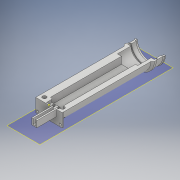
# Autodesk Inventor part: ExtendedHousingSide2wWireSupport
Saved by Autodesk Inventor 2019 (Build 230136000, 136)
## iProperties
Created: 2017-03-28
Part Number: ExtendedHousingSide2wWireSupport
Material: Generic
Document SubType Name: Modeling
Designer: Joseph
Density: 1 g/cm^3
Appearance: Default
Author: Joseph
Autodesk Inventor part; units mm, degrees
ref_plane "YZ Plane" through (0, 0, 0) normal (1, 0, 0) x (0, 1, 0)
ref_plane "XZ Plane" through (0, 0, 0) normal (0, 1, 0) x (-1, 0, 0)
sketch "Sketch1" plane through (0, 0, 0) normal (0, 1, 0) x (-1, 0, 0)
  circle A0 centre (0, 0) radius 19.05
  dimension "d0" = 38.1
  constraints: 1 centre point, 1 coincident
  measures "d0" diameter of A0
extrude "Extrusion1" add sketch "Sketch1" along normal blind 2
sketch "Sketch2" plane through (0, 2, 0) normal (0, 1, 0) x (1, 0, 0)
  circle A0 centre (0, 0) radius 19.05 projected
  line L0 (-8.575, -9) -> (-8.575, 9)
  line L1 (-8.575, 9) -> (11.425, 9)
  line L2 (11.425, 9) -> (11.425, -9)
  line L3 (11.425, -9) -> (-8.575, -9)
  dimension "d3" = 18
  dimension "d4" = 9
  dimension "d5" = 20
  dimension "d6" = 8.575
  constraints: 8 end point, 3 perpendicular, 1 vertical
  measures "d3" distance between parallel lines of L1 L3
  measures "d4" distance from line of point (0, 0) L3
  measures "d5" distance between parallel lines of L2 L0
  measures "d6" distance from line of point (0, 0) L0
extrude "Extrusion2" add sketch "Sketch2" along normal blind 130.5814
sketch "Sketch3" plane through (0, 132.5814, 0) normal (0, 1, 0) x (1, 0, 0)
  line L0 (-8.575, 9) -> (11.425, 9) projected
  line L1 (11.425, 9) -> (11.425, -9) projected
  line L2 (11.425, -9) -> (-8.575, -9) projected
  line L3 (-8.575, -9) -> (-8.575, 9) projected
  circle A0 centre (0, 0) radius 19.05 projected
  line L4 (11.425, 9) -> (11.425, -9) projected
  circle A1 centre (0, 0) radius 14.5441
  constraints: 1 coincident, 3 other
extrude "Extrusion3" cut sketch "Sketch3" against normal blind 20 contours L3 L2 A1 L0 | A1 L1
sketch "Sketch4" plane through (0, 2, 0) normal (0, 1, 0) x (1, 0, 0)
  line L0 (11.425, 9) -> (-8.575, 9) projected
  line L1 (-8.575, 9) -> (-8.575, -9) projected
  line L2 (-8.575, -9) -> (11.425, -9) projected
  line L3 (11.425, -9) -> (11.425, 9) projected
  line L4 (-8.575, -9) -> (11.425, -9) projected
  line L5 (-8.575, 9) -> (-8.575, -9) projected
  line L6 (11.425, 9) -> (-8.575, 9) projected
  arc A0 (11.425, 9) -> (11.425, -9) centre (0, 0) ccw projected
  line L7 (11.425, -9) -> (11.425, 9) projected
  arc A1 (11.425, -9) -> (11.425, 9) centre (0, 0) ccw projected
  circle A2 centre (0, 0) radius 14.5441 projected
  circle A3 centre (0, 0) radius 19.05 projected
  line L8 (5.565, -9) -> (5.565, -4.075)
  line L9 (5.565, -4.075) -> (-4.975, -4.075)
  line L10 (-4.975, -4.075) -> (-4.975, 4.075)
  line L11 (-4.975, 4.075) -> (5.565, 4.075)
  line L12 (5.565, 4.075) -> (5.565, 9)
  line L13 (-8.575, 9) -> (5.565, 9)
  line L14 (-8.575, -9) -> (-8.575, 9)
  line L15 (5.565, -9) -> (-8.575, -9)
  dimension "d11" = 14.14
  dimension "d12" = 3.6
  dimension "d13" = 8.15
  dimension "d14" = 4.075
  constraints: 16 end point, 4 point on line, 3 perpendicular, 2 collinear, 2 vertical
  measures "d11" distance between parallel lines of L1 L8
  measures "d12" distance between parallel lines of L1 L10
  measures "d13" distance between parallel lines of L11 L9
  measures "d14" distance from line of point (0, 0) L11
extrude "Extrusion4" add sketch "Sketch4" along normal blind 8.75 contours L12 L11 L10 L9 L8 L2 L1 L0
sketch "Sketch5" plane through (0, 0, 0) normal (0, 0, 1) x (1, 0, 0)
  circle A0 centre (0, 6.5) radius 2
  line L0 (5.565, 2) -> (-4.975, 2) projected
  point P0 (0, 0)
  dimension "d17" = 4
  dimension "d18" = 4.5
  constraints: 1 centre point
  measures "d17" diameter of A0
  measures "d18" distance from line of L0 A0.centre
extrude "Extrusion5" cut sketch "Sketch5" along normal blind 25.4 and the other way blind 25.4
sketch "Sketch6" plane through (0, 0, 0) normal (0, 0, 1) x (1, 0, 0)
  circle A0 centre (-13.05, 6.5) radius 2
  circle A1 centre (13.05, 6.5) radius 2
  line L0 (-19.05, 0) -> (19.05, 0) projected
  point P0 (0, 0)
  dimension "d23" = 4
  dimension "d24" = 4
  dimension "d25" = 6.5
  dimension "d26" = 6.5
  dimension "d27" = 6
  dimension "d28" = 6
  constraints: 2 centre point
  measures "d23" diameter of A0
  measures "d24" diameter of A1
  measures "d25" distance from line of L0 A0.centre
  measures "d26" distance from line of L0 A1.centre
  measures "d27" horizontal distance of L0.start A0.centre
  measures "d28" horizontal distance of L0.end A1.centre
extrude "Extrusion6" cut sketch "Sketch6" along normal mid plane 38.1
sketch "Sketch7" plane through (0, 2, 0) normal (0, 1, 0) x (1, 0, 0)
  line L0 (5.565, 9) -> (5.565, 4.075) projected
  line L1 (5.565, 4.075) -> (-4.975, 4.075) projected
  line L2 (-4.975, 4.075) -> (-4.975, -4.075) projected
  line L3 (-4.975, -4.075) -> (5.565, -4.075) projected
  line L4 (5.565, -4.075) -> (5.565, -9) projected
  line L5 (5.565, -9) -> (11.425, -9) projected
  line L6 (11.425, -9) -> (11.425, 9) projected
  line L7 (11.425, 9) -> (5.565, 9) projected
  line L8 (5.565, -6.5) -> (8.315, -6.5)
  line L9 (8.315, -6.5) -> (8.315, 6.5)
  line L10 (8.315, 6.5) -> (5.565, 6.5)
  line L11 (5.565, 6.5) -> (5.565, -6.5)
  point P0 (0, 0)
  dimension "d31" = 0
  dimension "d32" = 13
  dimension "d33" = 6.5
  dimension "d34" = 2.75
  constraints: 8 end point, 2 parallel, 1 horizontal, 1 perpendicular
  measures "d31" distance between parallel lines of L0 L11
  measures "d32" distance between parallel lines of L10 L8
  measures "d33" distance from line of point (0, 0) L10
  measures "d34" distance between parallel lines of L11 L9
extrude "Extrusion7" cut sketch "Sketch7" against normal blind 25.4 contours L10 L9 L8 L4 L11 L0
sketch "Sketch8" plane through (0, 132.5814, 0) normal (0, 1, 0) x (1, 0, 0)
  circle A0 centre (0, 0) radius 19.05
  circle A1 centre (0, 0) radius 21.5
  dimension "d37" = 43
  constraints: 2 centre point, 2 coincident
  measures "d37" diameter of A1
extrude "Extrusion8" add sketch "Sketch8" along normal blind 3.81 and the other way blind 3
chamfer "Chamfer1" distance 2.45 angle 45 1 edges at (-19.05, 129.5814, 0)
sketch "Sketch9" plane through (0, 136.3914, 0) normal (0, 1, 0) x (1, 0, 0)
  circle A0 centre (0, 0) radius 19.05 projected
  circle A1 centre (0, 0) radius 21.5 projected
  circle A2 centre (0, 0) radius 17.78
  circle A3 centre (0, 0) radius 20.5
  dimension "d45" = 35.56
  dimension "d46" = 41
  constraints: 2 centre point, 2 coincident
  measures "d45" diameter of A2
  measures "d46" diameter of A3
extrude "Extrusion9" add sketch "Sketch9" along normal blind 6.35 contours A0 | A3
sketch "Sketch10" plane through (0, 142.7414, 0) normal (0, 1, 0) x (1, 0, 0)
  circle A0 centre (0, 0) radius 17.78 projected
  circle A1 centre (0, 0) radius 20.5 projected
  circle A2 centre (0, 0) radius 21.5
  circle A3 centre (0, 0) radius 19.05
  dimension "d49" = 38.1
  constraints: 2 centre point, 2 coincident
  measures "d49" diameter of A3
extrude "Extrusion10" add sketch "Sketch10" along normal blind 3 contours A1 | A2
sketch "Sketch11" plane through (0, 136.3914, 0) normal (0, 1, 0) x (1, 0, 0)
  circle A0 centre (0, 0) radius 20.5 projected
  circle A1 centre (0, 0) radius 21.5 projected
extrude "Extrusion11" cut sketch "Sketch11" against normal blind 3.81
sketch "Sketch12" plane through (0, 145.7414, 0) normal (0, 1, 0) x (1, 0, 0)
  circle A0 centre (0, 0) radius 19.05 projected
  circle A1 centre (0, 0) radius 21.5 projected
  circle A2 centre (0, 0) radius 19.05 projected
  line L0 (-19.0352, -0.7504) -> (-21.4869, -0.7504)
  circle A3 centre (0, 0) radius 21.5 projected
  circle A4 centre (0, 0) radius 19.05 projected
  line L1 (-19.0352, 0.7496) -> (-21.4869, 0.7496)
  arc A5 (-21.4869, 0.7496) -> (-21.4869, -0.7504) centre (0, 0) ccw
  arc A6 (-19.0352, 0.7496) -> (-19.0352, -0.7504) centre (0, 0) ccw
  line L2 (-21.0034, -0.7504) -> (-16.8574, -0.7504)
  line L3 (-16.8574, -0.7504) -> (-16.8574, 0.7496)
  line L4 (-16.8574, 0.7496) -> (-21.0034, 0.7496)
  line L5 (-21.0034, 0.7496) -> (-21.0034, -0.7504)
  point P0 (-22.5185, -0.0004)
  dimension "d60" = 1.5
  dimension "d62" = 0.75
  constraints: 12 end point, 8 point on circle, 3 parallel, 2 centre point, 1 horizontal, 1 perpendicular, 1 point on line, 6 other
  measures "d60" distance between parallel lines of L1 L0
  measures "d62" distance from line of L1 point (-22.519, 0)
extrude "Extrusion12" cut sketch "Sketch12" against normal blind 11.1 contours L4 L3 L2 A0 | A0 L0 L5 L1 | L5 L0 A1 L1 picked at (-17.5877, -0.0838)
pattern_circular "Circular Pattern1" count 4 over 360 about axis through (0, 132.5814, 0) along (0, -1, 0) of "Extrusion12"
sketch "Sketch13" plane through (0, 132.5814, 0) normal (0, 1, 0) x (1, 0, 0)
  circle A0 centre (0, 0) radius 14.5441 projected
  circle A1 centre (0, 0) radius 19.05 projected
extrude "Extrusion13" cut sketch "Sketch13" against normal blind 0.5
sketch "Sketch14" plane through (0, 2, 0) normal (0, 1, 0) x (1, 0, 0)
  line L0 (5.565, -4.075) -> (5.565, 4.075) projected
  line L1 (5.565, 4.075) -> (-4.975, 4.075) projected
  line L2 (-4.975, 4.075) -> (-4.975, -4.075) projected
  line L3 (-4.975, -4.075) -> (5.565, -4.075) projected
  point P0 (0, 0)
extrude "Extrusion14" cut sketch "Sketch14" against normal blind 0.5
sketch "Sketch15" plane through (0, 132.5814, 0) normal (0, 1, 0) x (1, 0, 0)
  circle A0 centre (0, 0) radius 21.5 projected
  circle A1 centre (0, 0) radius 20.5 projected
extrude "Extrusion15" cut sketch "Sketch15" along normal blind 11.525
chamfer "Chamfer4" distance 1 angle 45 5 edges at (-20.5, 132.5814, 0) (-14.496, 144.1064, -14.4954) (14.4954, 144.1064, -14.496) (-14.4954, 144.1064, 14.496) (14.496, 144.1064, 14.4954)
fillet "Fillet1" radius 2 1 edges at (11.425, 7.6659, 0)
fillet "Fillet2" radius 2 1 edges at (11.425, 5.3341, 0)
sketch "Sketch16" plane through (0, 0, 0) normal (0, 0, 1) x (1, 0, 0)
  line L0 (-40.863, -42.6693) -> (49.311, -42.6693)
  line L1 (49.311, -42.6693) -> (49.311, 181.5634)
  line L2 (49.311, 181.5634) -> (-40.863, 181.5634)
  line L3 (-40.863, 181.5634) -> (-40.863, -42.6693)
  point P0 (0, 0)
  constraints: 8 end point, 2 parallel, 1 horizontal, 1 perpendicular
extrude "Extrusion16" cut sketch "Sketch16" along normal blind 25.4
chamfer "Chamfer5" distance 1.5 angle 45 2 edges at (-4.975, 10.75, -2.0375) (0.295, 10.75, -4.075)
ref_plane "Work Plane1" through (-4.975, 1.5, -23.125) normal (0, 0, 1) x (1, 0, 0)
sketch "Sketch17" plane through (-4.975, 1.5, -23.125) normal (0, 0, 1) x (1, 0, 0)
  line L0 (6.975, 5) -> (8.925, 5)
  line L1 (5.975, 6.7321) -> (6.95, 8.4208)
  line L2 (6.95, 8.4208) -> (8.925, 5)
  line L3 (3, 8.4208) -> (6.95, 8.4208)
  line L4 (1.025, 5) -> (3, 8.4208)
  line L5 (3, 1.5792) -> (1.025, 5)
  line L6 (6.95, 1.5792) -> (3, 1.5792)
  line L7 (8.925, 5) -> (6.95, 1.5792)
  line L8 (8.925, 5) -> (6.95, 1.5792)
  line L9 (3, 1.5792) -> (1.025, 5)
  line L10 (3, 8.4208) -> (6.95, 8.4208)
  line L11 (3, 8.4208) -> (1.025, 5)
  line L12 (6.95, 8.4208) -> (8.925, 5)
  circle A0 centre (4.975, 5) radius 2
  line L13 (8.925, 5) -> (6.95, 8.4208)
  point P0 (4.975, -1.5)
  dimension "d85" = 3.95
  dimension "d86" = 3.95
  dimension "d89" = 360
  constraints: 28 end point, 6 point on line, 2 horizontal, 1 coincident, 1 horizontal alignment, 24 other
  measures "d85" distance of point (4.975, 5) L0.end
  measures "d86" distance of point (4.975, 5) L1.end
extrude "Extrusion17" cut sketch "Sketch17" along normal blind 6 contours A0 L1 L2 L0 | L0 L7 L6 L5 L4 L3 L1 A0
sketch "Sketch18" plane through (0, 0, 0) normal (0, -1, 0) x (1, 0, 0)
  point P0 (0, 0)
sketch "Sketch19" plane through (0, 0, 0) normal (0, -1, 0) x (1, 0, 0)
  line L0 (3.19, 0.5) -> (3.19, -9)
  line L1 (8.315, 0) -> (11.425, 0) projected
  line L2 (10.69, 0) -> (10.69, -9)
  line L3 (10.69, -9) -> (3.19, -9)
  line L4 (5.565, -6.5) -> (5.565, 0) projected
  line L5 (8.315, 0) -> (8.315, -6.5) projected
  line L6 (-4.975, 0) -> (5.565, 0) projected
  line L7 (3.19, 0) -> (5.565, 0)
  line L8 (5.565, -9) -> (5.565, -6.5) projected
  line L9 (5.565, 0) -> (5.565, -6.5)
  line L10 (5.565, -6.5) -> (8.315, -6.5)
  line L11 (8.315, 0) -> (10.69, 0)
  point P0 (0, 0)
  dimension "d93" = 2.375
  dimension "d94" = 2.375
  dimension "d95" = 9.5
  constraints: 14 end point, 3 perpendicular, 3 point on line, 2 vertical, 1 collinear, 1 parallel
  measures "d93" distance between parallel lines of L4 L0
  measures "d94" distance between parallel lines of L2 L5
  measures "d95" distance of L0.end L0.start
extrude "Extrusion18" add sketch "Sketch19" along normal blind 28
sketch "Sketch20" plane through (0, -28, 0) normal (0, -1, 0) x (1, 0, 0)
  line L0 (5.19, 0.0001) -> (5.19, -7)
  line L1 (8.69, 0) -> (8.69, -7)
  line L2 (8.69, -7) -> (5.19, -7)
  line L3 (3.19, 0) -> (3.19, -9) projected
  line L4 (10.69, -9) -> (10.69, 0) projected
  line L5 (3.19, -9) -> (10.69, -9) projected
  line L6 (5.19, 0.0001) -> (5.565, 0.0001)
  line L7 (5.565, -6.5) -> (8.315, -6.5) projected
  line L8 (5.565, 0.0001) -> (5.565, -6.5)
  line L9 (5.565, -6.5) -> (8.315, -6.5)
  line L10 (8.315, -6.5) -> (8.315, 0) projected
  line L11 (8.315, -6.5) -> (8.315, 0)
  line L12 (8.315, 0) -> (8.69, 0)
  point P0 (0, 0)
  dimension "d98" = 2
  dimension "d99" = 2
  dimension "d101" = 2
  constraints: 16 end point, 4 perpendicular, 2 vertical, 1 collinear, 1 horizontal
  measures "d98" distance between parallel lines of L0 L3
  measures "d99" distance between parallel lines of L4 L1
  measures "d101" distance between parallel lines of L5 L2
extrude "Extrusion19" cut sketch "Sketch20" against normal blind 52
sketch "Sketch21" plane through (0, 0, 0) normal (0, -1, 0) x (1, 0, 0)
  arc A0 (-19.05, 0) -> (19.05, 0) centre (0, 0) ccw projected
  line L0 (-19.05, 0) -> (19.05, 0)
  line L1 (19.05, 0) -> (19.05, -19.05)
  line L2 (19.05, -19.05) -> (-19.05, -19.05)
  line L3 (-19.05, -19.05) -> (-19.05, 0)
  point P0 (0, -19.05)
  constraints: 8 end point, 2 parallel, 1 horizontal, 1 midpoint, 1 perpendicular, 1 point on circle, 1 point on line
extrude "Extrusion20" add sketch "Sketch21" against normal blind 2 contours A0 L2 L3 | A0 L1 L2
sketch "Sketch22" plane through (0, 2, 0) normal (0, 1, 0) x (1, 0, 0)
  circle A0 centre (16.05, 16.05) radius 1.651
  line L0 (19.05, 0) -> (19.05, 19.05) projected
  line L1 (19.05, 19.05) -> (0, 19.05) projected
  circle A1 centre (-16.4497, 16.05) radius 1.651
  point P0 (0, 0)
  dimension "d106" = 3.302
  dimension "d107" = 3
  dimension "d108" = 3
  dimension "d109" = 3.302
  constraints: 2 centre point
  measures "d106" diameter of A0
  measures "d107" distance from line of A0.centre L0
  measures "d108" distance from line of A0.centre L1
  measures "d109" diameter of A1
extrude "Extrusion21" cut sketch "Sketch22" against normal through all
sketch "Sketch23" plane through (-8.575, 112.5814, -9) normal (0, 0, 1) x (1, 0, 0)
  line L0 (0, -101.8314) -> (0, 0) projected
  line L1 (20, -102.099) -> (20, 0) projected
  line L2 (0, -101.8314) -> (20, -101.8314)
  line L3 (20, -101.8314) -> (20, 0)
  line L4 (20, 0) -> (0, 0)
  line L5 (0, 0) -> (0, -101.8314)
  point P0 (8.575, -112.5814)
  constraints: 8 end point, 2 parallel, 1 horizontal, 1 perpendicular
extrude "Extrusion22" cut sketch "Sketch23" against normal blind 1
sketch "Sketch24" plane through (0, 0, 0) normal (0, 0, 1) x (1, 0, 0)
  circle A0 centre (-13.05, 6.5) radius 2 projected
  circle A1 centre (-13.05, 6.5) radius 2.75
  arc A2 (13.2375, 4.5088) -> (13.2375, 8.4912) centre (13.05, 6.5) ccw projected
  circle A3 centre (13.05, 6.5) radius 2.75
  point P0 (0, 0)
  dimension "d114" = 5.5
  dimension "d115" = 5.5
  constraints: 2 centre point, 2 coincident
  measures "d114" diameter of A1
  measures "d115" diameter of A3
extrude "Extrusion23" cut sketch "Sketch24" against normal through all contours A0 | A1 | A3
ref_plane "Work Plane2" through (0, 0, -19.05) normal (0, 0, -1) x (-1, 0, 0)
sketch "Sketch25" plane through (0, 0, -19.05) normal (0, 0, -1) x (-1, 0, 0)
  circle A0 centre (0, 6.5) radius 2 projected
  line L0 (-2.3094, 10.5) -> (2.3094, 10.5)
  line L1 (2.3094, 10.5) -> (4.6188, 6.5)
  line L2 (4.6188, 6.5) -> (2.3094, 2.5)
  line L3 (2.3094, 2.5) -> (-2.3094, 2.5)
  line L4 (-2.3094, 2.5) -> (-4.6188, 6.5)
  line L5 (-4.6188, 6.5) -> (-2.3094, 10.5)
  point P0 (0, 0)
  dimension "d118" = 4
  constraints: 12 end point, 1 coincident, 1 horizontal, 13 other
  measures "d118" distance from line of L0 point (0, 6.5)
extrude "Extrusion24" cut sketch "Sketch25" against normal up to surface (1.925 mm away)
body "Solid1"
